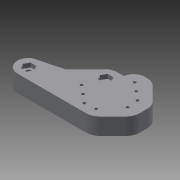
# Autodesk Inventor part: joint1+ax12imprint+v2
Saved by Autodesk Inventor 2014 (Build 180170000, 170)
## iProperties
Created: 2014-01-13
Part Number: joint1+ax12imprint+v2
Material: Générique
Document SubType Name: Modeling
Designer: helly
Density: 1 g/cm^3
Appearance: Par défaut
Author: helly
Autodesk Inventor part; units mm, degrees
ref_plane "YZ Plane" through (0, 0, 0) normal (1, 0, 0) x (0, 1, 0)
ref_plane "XZ Plane" through (0, 0, 0) normal (0, 1, 0) x (-1, 0, 0)
ref_plane "XY Plane" through (0, 0, 0) normal (0, 0, 1) x (1, 0, 0)
sketch "Esquisse1" plane through (0, 0, 0) normal (0, 0, 1) x (1, 0, 0)
  line L0 (0, 0) -> (52, 0) construction
  line L1 (0, 0) -> (27.5772, 27.5772) construction
  circle A0 centre (27.5772, 27.5772) radius 2
  circle A1 centre (0, 0) radius 2
  line L2 (0, 0) -> (0, -8) construction
  line L3 (0, 0) -> (-5.6569, 5.6569) construction
  line L4 (68.2971, -8) -> (-19.3137, -8)
  line L5 (27.5772, 27.5772) -> (27.5772, 35.5772) construction
  line L6 (-19.3137, -8) -> (24.2635, 35.5772)
  line L7 (24.2635, 35.5772) -> (68.2971, 35.5772)
  line L8 (27.5772, 27.5772) -> (49, 27.5772) construction
  line L9 (27.5772, 27.5772) -> (55.1548, 4.4368) construction
  line L10 (27.5772, 27.5772) -> (36.2548, 37.9188) construction
  line L11 (36.2548, 37.9188) -> (41.2341, 33.7406) construction
  line L12 (41.2341, 33.7406) -> (47.3624, 28.5983) construction
  line L13 (47.3624, 28.5983) -> (53.4908, 23.456) construction
  line L14 (53.4908, 23.456) -> (59.6192, 18.3137) construction
  line L15 (55.1548, 4.4368) -> (60.2971, 10.5652) construction
  circle A2 centre (41.2341, 33.7406) radius 1 construction
  circle A3 centre (47.3624, 28.5983) radius 1
  circle A4 centre (53.4908, 23.456) radius 1
  circle A5 centre (59.6192, 18.3137) radius 1
  circle A6 centre (60.2971, 10.5652) radius 1
  circle A7 centre (23.8788, 13.0574) radius 1 construction
  circle A8 centre (30.0072, 7.9151) radius 1
  circle A9 centre (36.1355, 2.7728) radius 1
  circle A10 centre (42.2639, -2.3695) radius 1
  circle A11 centre (50.0125, -1.6915) radius 1
  line L16 (60.2971, 10.5652) -> (68.2971, 10.5652) construction
  line L17 (68.2971, 35.5772) -> (68.2971, -8)
  dimension "d39" = 39
  dimension "d41" = 4
  dimension "d44" = 8
  dimension "d64" = 8
  dimension "d80" = 45
  dimension "d82" = 8
  dimension "d101" = 36
  dimension "d102" = 40
  dimension "d103" = 13.5
  dimension "d104" = 6.5
  dimension "d105" = 8
  dimension "d106" = 8
  dimension "d107" = 8
  dimension "d108" = 8
  dimension "d109" = 2
  dimension "d110" = 8
  constraints: 36 end point, 12 centre point, 10 perpendicular, 7 coincident, 5 equal radius, 5 symmetric about line, 4 point on line, 3 collinear, 2 parallel, 1 horizontal, 5 other
  measures "d39" distance of L0.start L1.end
  measures "d41" diameter of A0
  measures "d44" distance of L2.start L2.end
  measures "d64" distance of L2.start L3.end
  measures "d80" angle of L0 L1
  measures "d82" distance of L5.start L5.end
  measures "d101" distance of L5.start L9.end
  measures "d102" angle of L8 L9
  measures "d103" distance of L5.start L10.end
  measures "d104" distance of L10.end L11.end
  measures "d105" distance of L11.end L12.end
  measures "d106" distance of L12.end L13.end
  measures "d107" distance of L13.end L14.end
  measures "d108" distance of L9.end L15.end
  measures "d109" diameter of A2
  measures "d110" distance of L16.start L16.end
extrude "Extrusion15" add sketch "Esquisse1" along normal blind 12
sketch "Esquisse13" plane through (0, 0, 12) normal (0, 0, 1) x (1, 0, 0)
  circle A0 centre (0, 0) radius 2 projected
  circle A1 centre (27.5772, 27.5772) radius 2 projected
  line L0 (68.2971, -8) -> (68.2971, 35.5772) projected
  line L1 (68.2971, 35.5772) -> (24.2635, 35.5772) projected
  line L2 (24.2635, 35.5772) -> (-19.3137, -8) projected
  circle A2 centre (27.5772, 27.5772) radius 12 construction
  line L3 (39.5772, 35.5772) -> (39.5772, 27.5772)
  line L4 (0, 0) -> (0, 8) construction
  line L5 (-4.4796, 6.8341) -> (30.5997, 15.964)
  arc A3 (30.5997, 15.964) -> (39.5772, 27.5772) centre (27.5772, 27.5772) ccw
  dimension "d128" = 24
  dimension "d129" = 8
  constraints: 6 end point, 4 point on circle, 3 point on line, 2 centre point, 2 coincident, 2 parallel, 2 tangent
  measures "d128" diameter of A2
  measures "d129" distance of L4.start L4.end
extrude "Extrusion16" cut sketch "Esquisse13" against normal blind 7 contours L3 A3 L5 L2 L1
sketch "Esquisse14" plane through (0, 0, 12) normal (0, 0, 1) x (1, 0, 0)
  line L0 (-19.3137, -8) -> (68.2971, -8) projected
  circle A0 centre (0, 0) radius 2 projected
  line L1 (4.0415, 0) -> (2.0207, -3.5)
  line L2 (2.0207, -3.5) -> (-2.0207, -3.5)
  line L3 (-2.0207, -3.5) -> (-4.0415, 0)
  line L4 (-4.0415, 0) -> (-2.0207, 3.5)
  line L5 (-2.0207, 3.5) -> (2.0207, 3.5)
  line L6 (2.0207, 3.5) -> (4.0415, 0)
  line L7 (2.0207, 3.5) -> (2.0207, -3.5) construction
  dimension "d132" = 7
  constraints: 14 end point, 1 coincident, 1 parallel, 1 perpendicular, 13 other
  measures "d132" distance of L5.end L1.end
sketch "Esquisse15" plane through (0, 0, 5) normal (0, 0, 1) x (1, 0, 0)
  circle A0 centre (27.5772, 27.5772) radius 2 projected
  arc A1 (30.5997, 15.964) -> (39.5772, 27.5772) centre (27.5772, 27.5772) ccw projected
  line L0 (31.6186, 27.5772) -> (29.5979, 24.0772)
  line L1 (29.5979, 24.0772) -> (25.5564, 24.0772)
  line L2 (25.5564, 24.0772) -> (23.5357, 27.5772)
  line L3 (23.5357, 27.5772) -> (25.5564, 31.0772)
  line L4 (25.5564, 31.0772) -> (29.5979, 31.0772)
  line L5 (29.5979, 31.0772) -> (31.6186, 27.5772)
  line L6 (-19.3137, -8) -> (68.2971, -8) projected
  line L7 (-2.0207, 3.5) -> (2.0207, 3.5) projected
  point P0 (0, 0)
  constraints: 12 end point, 2 parallel, 1 coincident, 13 other
extrude "Extrusion17" cut sketch "Esquisse14" against normal blind 3
extrude "Extrusion18" cut sketch "Esquisse15" against normal blind 3
fillet "Congé8" radius 8 1 edges at (-19.3137, -8, 6)
fillet "Congé9" radius 8 1 edges at (24.2635, 35.5772, 2.5)
fillet "Congé10" radius 8 1 edges at (39.5772, 35.5772, 8.5)
chamfer "Chanfrein1" distance 15 angle 45 1 edges at (68.2971, 35.5772, 6)
chamfer "Chanfrein2" distance 15 angle 45 1 edges at (68.2971, -8, 6)
fillet "Congé12" radius 10 1 edges at (53.2971, -8, 6)
fillet "Congé13" radius 10 1 edges at (68.2971, 7, 6)
fillet "Congé14" radius 10 1 edges at (68.2971, 20.5772, 6)
fillet "Congé15" radius 10 1 edges at (53.2971, 35.5772, 6)
